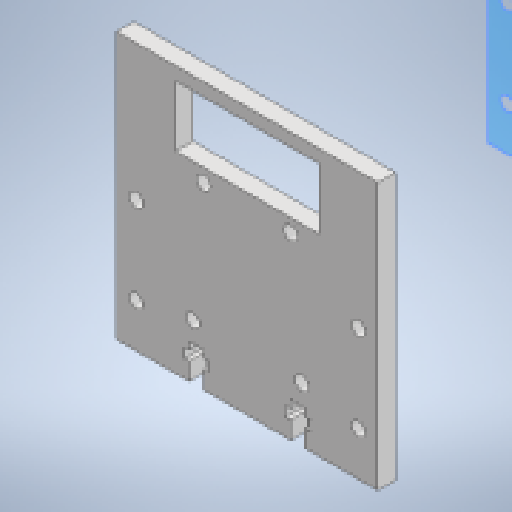
# Autodesk Inventor part: стена_для_рельс
Saved by Autodesk Inventor 2023.1 (Build 271208000, 208)
## iProperties
Created: 2026-02-04
Part Number: стена_для_рельс
Material: Типовые
Document SubType Name: Modeling
Designer: DELL
Density: 1 g/cm^3
Appearance: По умолчанию
Author: DELL
Autodesk Inventor part; units mm, degrees
ref_plane "YZ Plane" through (0, 0, 0) normal (1, 0, 0) x (0, 1, 0)
ref_plane "XZ Plane" through (0, 0, 0) normal (0, 1, 0) x (-1, 0, 0)
ref_plane "XY Plane" through (0, 0, 0) normal (0, 0, 1) x (1, 0, 0)
sketch "Эскиз1" plane through (0, 0, 0) normal (0, 0, 1) x (1, 0, 0)
  line L0 (-30, 21.6) -> (30, 21.6)
  line L1 (30, 21.6) -> (30, -21.6)
  line L2 (30, -21.6) -> (-30, -21.6)
  line L3 (-30, -21.6) -> (-30, 21.6)
  line L4 (-30, 21.6) -> (30, -21.6) construction
  line L5 (30, 21.6) -> (-30, -21.6) construction
  point P0 (0, 0)
  dimension "d0" = 60
  dimension "d1" = 43.2
  constraints: 12 end point, 2 midpoint, 2 parallel, 1 horizontal, 1 perpendicular
  measures "d0" distance of L1.end L2.end
  measures "d1" distance of L0.end L1.end
extrude "Выдавливание1" add sketch "Эскиз1" along normal blind 4
sketch "Эскиз2" plane through (0, 0, 0) normal (0, 0, -1) x (-1, 0, 0)
  line L0 (-12.5, -9) -> (12.5, -9) construction
  line L1 (0, 0) -> (0, -21.6) construction
  line L2 (30, -21.6) -> (-30, -21.6) projected
  circle A0 centre (-12.5, -9) radius 1.6
  circle A1 centre (12.5, -9) radius 1.6
  line L3 (-30, -21.6) -> (-30, 21.6) projected
  line L4 (-30, 0) -> (30, 0) construction
  line L5 (30, 21.6) -> (30, -21.6) projected
  point P0 (0, -9)
  dimension "d4" = 25
  dimension "d5" = 3.2
  dimension "d6" = 3.2
  dimension "d7" = 9
  constraints: 6 end point, 4 midpoint, 2 centre point, 2 coincident, 1 horizontal, 1 point on line
  measures "d4" distance of L0.start L0.end
  measures "d5" diameter of A0
  measures "d6" diameter of A1
  measures "d7" distance between parallel lines of L4 L0
extrude "Выдавливание2" cut sketch "Эскиз2" against normal blind 4
sketch "Эскиз3" plane through (0, 0, 0) normal (0, 0, -1) x (-1, 0, 0)
  circle A0 centre (-25.5, 8.4) radius 1.75 construction
  circle A1 centre (25.5, 8.4) radius 1.75 construction
  circle A2 centre (25.5, -11.6) radius 1.75 construction
  circle A3 centre (-25.5, -11.6) radius 1.75 construction
  circle A4 centre (-25.5, 8.4) radius 1.6
  circle A5 centre (25.5, 8.4) radius 1.6
  circle A6 centre (-25.5, -11.6) radius 1.6
  circle A7 centre (25.5, -11.6) radius 1.6
  point P0 (0, 0)
  dimension "d10" = 3.2
  dimension "d11" = 3.2
  dimension "d12" = 3.2
  dimension "d13" = 3.2
  constraints: 4 centre point, 4 coincident
  measures "d10" diameter of A4
  measures "d11" diameter of A5
  measures "d12" diameter of A6
  measures "d13" diameter of A7
extrude "Выдавливание3" cut sketch "Эскиз3" against normal blind 10
sketch "Эскиз4" plane through (0, 0, 0) normal (0, 0, -1) x (-1, 0, 0)
  line L0 (-30, 21.6) -> (30, 21.6) construction
  line L1 (-30, 21.6) -> (30, 21.6) projected
  line L2 (-30, 21.6) -> (30, 21.6)
  line L3 (30, 21.6) -> (30, 39.6)
  line L4 (30, 39.6) -> (-30, 39.6)
  line L5 (-30, 39.6) -> (-30, 21.6)
  dimension "d18" = 60
  dimension "d19" = 18
  constraints: 8 end point, 2 parallel, 1 horizontal, 1 perpendicular
  measures "d18" distance of L4.end L3.end
  measures "d19" distance of L3.end L2.end
extrude "Выдавливание4" add sketch "Эскиз4" against normal blind 4
sketch "Эскиз5" plane through (0, 0, 0) normal (0, 0, -1) x (-1, 0, 0)
  line L0 (-11.55, 23.6) -> (11.45, 23.6) construction
  line L1 (11.45, 23.6) -> (11.45, 35.6) construction
  line L2 (-11.55, 23.6) -> (11.45, 35.6) construction
  line L3 (-16.55, 36.6) -> (16.45, 36.6)
  line L4 (16.45, 36.6) -> (16.45, 22.6)
  line L5 (16.45, 22.6) -> (-16.55, 22.6)
  line L6 (-16.55, 22.6) -> (-16.55, 36.6)
  line L7 (-16.55, 36.6) -> (16.45, 22.6) construction
  line L8 (16.45, 36.6) -> (-16.55, 22.6) construction
  point P0 (0, 0)
  point P1 (-0.05, 29.6)
  dimension "d22" = 1
  dimension "d23" = 5
  constraints: 18 end point, 3 midpoint, 2 horizontal, 2 parallel, 1 perpendicular, 1 vertical, 3 other
  measures "d22" distance between parallel lines of L5 L0
  measures "d23" distance between parallel lines of L4 L1
extrude "Выдавливание5" cut sketch "Эскиз5" against normal blind 4
sketch "Эскиз6" plane through (0, 0, 4) normal (0, 0, 1) x (1, 0, 0)
  line L0 (11.7, 17.6) -> (11.7, 21.6) construction
  line L1 (11.7, 21.6) -> (30, 21.6) construction
  line L2 (30, 21.6) -> (30, 17.6) construction
  line L3 (30, 17.6) -> (11.7, 17.6) construction
  line L4 (-8.3, 17.6) -> (-8.3, 21.6) construction
  line L5 (-8.3, 21.6) -> (8.3, 21.6) construction
  line L6 (8.3, 21.6) -> (8.3, 17.6) construction
  line L7 (8.3, 17.6) -> (-8.3, 17.6) construction
  line L8 (-11.7, 21.6) -> (-11.7, 17.6) construction
  line L9 (-11.7, 17.6) -> (-30, 17.6) construction
  line L10 (-30, 17.6) -> (-30, 21.6) construction
  line L11 (-30, 21.6) -> (-11.7, 21.6) construction
  line L12 (11.7, 21.6) -> (8.3, 17.6) construction
  line L13 (-8.3, 21.6) -> (-11.7, 17.6) construction
  circle A0 centre (-10, 19.6) radius 1.6
  circle A1 centre (10, 19.6) radius 1.6
  point P0 (0, 0)
  dimension "d26" = 3.2
  dimension "d27" = 3.2
  constraints: 28 end point, 6 horizontal, 6 vertical, 2 centre point, 2 midpoint, 12 other
  measures "d26" diameter of A0
  measures "d27" diameter of A1
extrude "Выдавливание6" cut sketch "Эскиз6" against normal blind 10
sketch "Эскиз7" plane through (0, 0, 0) normal (0, 0, -1) x (-1, 0, 0)
  line L0 (-10, -21.6) -> (-13.3, -21.6)
  line L1 (-13.3, -21.6) -> (-13.3, -13.6)
  line L2 (-13.3, -13.6) -> (-10, -13.6)
  line L3 (-10, -13.6) -> (-10, -21.6)
  line L4 (-20, -21.6) -> (20, -21.6) projected
  line L5 (30, -21.6) -> (-30, -21.6) projected
  line L6 (-8.9, -17.6) -> (-14.4, -17.6)
  line L7 (-14.4, -17.6) -> (-14.4, -15.3)
  line L8 (-14.4, -15.3) -> (-8.9, -15.3)
  line L9 (-8.9, -15.3) -> (-8.9, -17.6)
  line L10 (-11.65, -13.6) -> (-11.65, -21.6) construction
  line L11 (0, -21.6) -> (0, -16.45)
  line L12 (10, -21.6) -> (13.3, -21.6)
  line L13 (13.3, -21.6) -> (13.3, -13.6)
  line L14 (13.3, -13.6) -> (10, -13.6)
  line L15 (10, -13.6) -> (10, -21.6)
  line L16 (8.9, -17.6) -> (14.4, -17.6)
  line L17 (14.4, -17.6) -> (14.4, -15.3)
  line L18 (14.4, -15.3) -> (8.9, -15.3)
  line L19 (8.9, -15.3) -> (8.9, -17.6)
  line L20 (11.65, -13.6) -> (11.65, -21.6) construction
  point P0 (0, 0)
  point P1 (-11.65, -15.3)
  point P2 (11.65, -15.3)
  point P3 (-13.3, -17.6)
  point P4 (-10, -17.6)
  point P5 (-10, -15.3)
  point P6 (-13.3, -15.3)
  point P7 (13.3, -15.3)
  point P8 (10, -15.3)
  point P9 (10, -17.6)
  point P10 (13.3, -17.6)
  dimension "d30" = 3.3
  dimension "d31" = 8
  dimension "d32" = 10
  dimension "d33" = 5.5
  dimension "d34" = 2.3
  dimension "d35" = 4
  constraints: 38 end point, 11 symmetric about line, 4 midpoint, 4 parallel, 3 point on line, 2 horizontal, 2 perpendicular, 2 vertical
  measures "d30" distance of L1.end L2.end
  measures "d31" distance of L2.end L0.start
  measures "d32" distance from line of L11.start L3
  measures "d33" distance of L7.end L8.end
  measures "d34" distance of L6.end L7.end
  measures "d35" distance between parallel lines of L4 L6
extrude "Выдавливание7" cut sketch "Эскиз7" against normal blind 4
